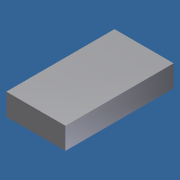
# Autodesk Inventor part: Inverter Standin
Saved by Autodesk Inventor 2012 (Build 160160000, 160)
## iProperties
Created: 2012-03-15
Part Number: Inverter Standin
Material: Default
Document SubType Name: Modeling
Designer: Ed
Mass: 4300 g
Surface Area: 2270.7 cm^2
Volume: 5287.83 cm^3
Density: 0.813188 g/cm^3
Author: Ed
Autodesk Inventor part; units mm, degrees
ref_plane "YZ Plane" through (0, 0, 0) normal (1, 0, 0) x (0, 1, 0)
ref_plane "XZ Plane" through (0, 0, 0) normal (0, 1, 0) x (-1, 0, 0)
ref_plane "XY Plane" through (0, 0, 0) normal (0, 0, 1) x (1, 0, 0)
sketch "Sketch1" plane through (0, 0, 0) normal (0, 0, 1) x (1, 0, 0)
  line L0 (0, 0) -> (199, 0)
  line L1 (199, 0) -> (199, 73)
  line L2 (199, 73) -> (0, 73)
  line L3 (0, 73) -> (0, 0)
  dimension "d0" = 73
  dimension "d1" = 199
  constraints: 8 end point, 2 parallel, 1 horizontal, 1 perpendicular
  measures "d0" distance of L2.end L0.start
  measures "d1" distance of L0.start L0.end
extrude "Extrusion1" add sketch "Sketch1" along normal blind 364
body "Solid1"
